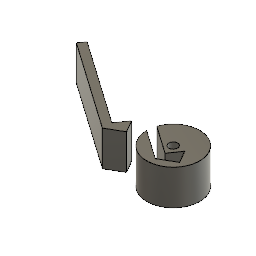
LoadShuttle v1 (Autodesk Fusion 360 design; units mm, degrees)
Autodesk Fusion 360 part; units mm, degrees
sketch "Sketch1" plane through (0, 0, 0) normal (0, 1, 0) x (1, 0, 0)
  circle A0 centre (0, 0) radius 15
  line L0 (-15, 0) -> (1.383, -11.4715)
  line L1 (-15, 0) -> (-5, 0) construction
  circle A1 centre (0, 0) radius 2.5
  line L2 (1.383, -11.4715) -> (10.0433, -6.4715)
  line L3 (1.383, -11.4715) -> (9.383, -11.4715) construction
  line L4 (10.0433, -6.4715) -> (6.0433, 0.4567)
  line L5 (6.0433, 0.4567) -> (1.4547, -6.0965)
  line L6 (6.0433, 0.4567) -> (14.0433, 0.4567) construction
  line L7 (1.4547, -6.0965) -> (-14.1912, 4.8589)
  dimension "d1" = 30
  dimension "d2" = 20
  dimension "d3" = 35
  dimension "d6" = 5
  dimension "d7" = 30
  dimension "d8" = 10
  dimension "d9" = 8
  dimension "d10" = 125
  dimension "d11" = 8
  constraint coincident A0.centre A1.centre
  constraint horizontal L1
  constraint coincident A0 L0.start
  constraint concentric A0 A1
  constraint horizontal L3
  constraint perpendicular L2 L4
  constraint horizontal L6
  constraint coincident A0 L7.end
  constraint perpendicular L5 L7
  measures "d1" diameter of A0
  measures "d2" distance of L0.start L0.end
  measures "d3" angle of L0 L1
  measures "d6" diameter of A1
  measures "d7" angle of L2 L3
  measures "d8" distance of L0.end L2.end
  measures "d9" distance of L2.end L4.end
  measures "d10" angle of L5 L6
  measures "d11" distance of L4.end L5.end
extrude "Extrude1" add sketch "Sketch1" along normal blind 20 contours A0 L0 L2 L4 L5 L7 picked at (10.3064, -2.7502) makes body 1
sketch "Sketch2" plane through (0, 0, 0) normal (0, 1, 0) x (1, 0, 0)
  circle A0 centre (0, 0) radius 2.5
  arc A1 (-15, 0) -> (-14.1912, 4.8589) centre (0, 0) ccw
  line L0 (-14.1912, 4.8589) -> (1.4547, -6.0965)
  line L1 (1.4547, -6.0965) -> (6.0433, 0.4567)
  line L2 (6.0433, 0.4567) -> (10.0433, -6.4715)
  line L3 (10.0433, -6.4715) -> (1.383, -11.4715)
  line L4 (1.383, -11.4715) -> (-15, 0)
  line L5 (-14.1912, 4.8589) -> (1.4547, -6.0965)
  line L6 (6.0433, 0.4567) -> (10.0433, -6.4715)
  line L7 (1.383, -11.4715) -> (-15, 0)
  line L8 (-15, 0) -> (-47.7661, 22.9431)
  line L9 (-47.7661, 22.9431) -> (-45.2171, 26.5834)
  line L10 (-14.1912, 4.8589) -> (-45.2171, 26.5834)
  line L11 (1.4547, -6.0965) -> (6.0433, 0.4567)
  line L12 (10.0433, -6.4715) -> (1.383, -11.4715)
  dimension "d14" = 40
  constraint coincident A1.end L0.start
  constraint coincident L0.end L1.start
  constraint coincident L1.end L2.start
  constraint coincident L2.end L3.start
  constraint coincident L3.end L4.start
  constraint coincident A1.start L4.end
  constraint parallel L7 L8
  constraint perpendicular L8 L9
  constraint perpendicular L9 L10
  measures "d14" distance of A1.start L8.end
extrude "Extrude2" add sketch "Sketch2" along normal blind 20 separate body contours L0 L1 L2 L3 L4 L5 L6 L7 L8 L9 L10 L11 L12 makes body 2
move_body "Move1" bodies 2 to x (1, 0, 0) y (0, 1, 0) z (0, 0, 1) at (-30, 0, 0)
